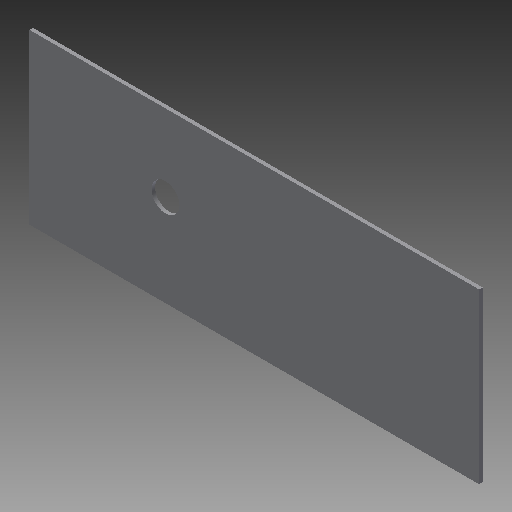
# Autodesk Inventor part: LFEV2017_TSI_003
Saved by Autodesk Inventor 2017 (Build 210142000, 142)
## iProperties
Created: 2017-04-03
Part Number: LFEV2017_TSI_003
Material: Generic
Document SubType Name: Modeling
Designer: hoeflinc
Density: 1 g/cm^3
Appearance: Default
Material_size: Aluminum     Thickness: .125"
Quantity: 1
Author: hoeflinc
Autodesk Inventor part; units mm, degrees
ref_plane "YZ Plane" through (0, 0, 0) normal (1, 0, 0) x (0, 1, 0)
ref_plane "XZ Plane" through (0, 0, 0) normal (0, 1, 0) x (-1, 0, 0)
ref_plane "XY Plane" through (0, 0, 0) normal (0, 0, 1) x (1, 0, 0)
sketch "Sketch1" plane through (0, 0, 0) normal (0, 0, 1) x (1, 0, 0)
  line L0 (0, 0) -> (406.4, 0)
  line L1 (406.4, 0) -> (406.4, 152.4)
  line L2 (406.4, 152.4) -> (0, 152.4)
  line L3 (0, 152.4) -> (0, 0)
  dimension "d0" = 152.4
  dimension "d1" = 406.4
  constraints: 8 end point, 2 parallel, 1 horizontal, 1 perpendicular
  measures "d0" distance of L2.end L0.start
  measures "d1" distance of L0.start L0.end
extrude "Extrusion1" add sketch "Sketch1" along normal blind 3.175
sketch "Sketch2" plane through (0, 0, 3.175) normal (0, 0, 1) x (1, 0, 0)
  circle A0 centre (123.0122, 82.804) radius 12.7
  line L0 (0, 152.4) -> (0, 0) projected
  line L1 (0, 0) -> (406.4, 0) projected
  dimension "d4" = 25.4
  dimension "d5" = 123.0122
  dimension "d6" = 82.804
  constraints: 1 centre point
  measures "d4" diameter of A0
  measures "d5" distance from line of A0.centre L0
  measures "d6" distance from line of A0.centre L1
extrude "Extrusion2" cut sketch "Sketch2" against normal blind 3.175
body "Solid1"
